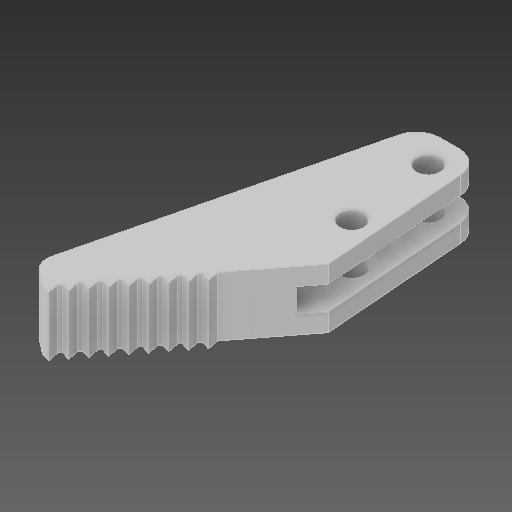
# Autodesk Inventor part: capit
Saved by Autodesk Inventor 2019 (Build 230136000, 136)
## iProperties
Created: 2016-12-05
Part Number: capit
Material: Generic
Document SubType Name: Modeling
Designer: MuhammadArdian
Density: 1 g/cm^3
Appearance: Default
Author: MuhammadArdian
Autodesk Inventor part; units mm, degrees
ref_plane "YZ Plane" through (0, 0, 0) normal (1, 0, 0) x (0, 1, 0)
ref_plane "XZ Plane" through (0, 0, 0) normal (0, 1, 0) x (-1, 0, 0)
sketch "Sketch1" plane through (0, 0, 0) normal (0, 1, 0) x (-1, 0, 0)
  line L0 (-38.3993, -26.9176) -> (-33.0009, -96.7091)
  line L1 (-33.0009, -96.7091) -> (-8.0012, -96.5869)
  circle A0 centre (-23.2715, -84.2034) radius 5
  circle A1 centre (-27.3538, -47.8392) radius 5
  line L2 (-38.3993, -26.9176) -> (16.6007, -26.9176) construction
  arc A2 (22.7463, 28.593) -> (19.9992, 36.438) centre (15.3555, 30.4084) ccw
  line L3 (-8.0012, -96.5869) -> (22.7463, 28.593)
  line L4 (11.975, 39.0871) -> (13.9695, 41.0816)
  line L5 (13.9695, 41.0816) -> (19.9992, 36.438)
  line L6 (13.9695, 41.0816) -> (16.437, 44.2856)
  line L7 (16.437, 44.2856) -> (13.9695, 41.0816)
  line L8 (13.9695, 41.0816) -> (10.2037, 42.2949)
  line L9 (10.2037, 42.2949) -> (11.1441, 37.4129)
  line L10 (10.3086, 36.328) -> (6.5427, 37.5413)
  line L11 (6.5427, 37.5413) -> (7.4831, 32.6592)
  line L12 (6.6476, 31.5743) -> (2.8817, 32.7876)
  line L13 (2.8817, 32.7876) -> (3.8221, 27.9055)
  line L14 (2.9866, 26.8207) -> (-0.7792, 28.034)
  line L15 (-0.7792, 28.034) -> (0.1612, 23.1519)
  line L16 (-0.6744, 22.067) -> (-4.4402, 23.2803)
  line L17 (-4.4402, 23.2803) -> (-3.4998, 18.3982)
  line L18 (-4.3353, 17.3133) -> (-8.1012, 18.5266)
  line L19 (-8.1012, 18.5266) -> (-7.1608, 13.6446)
  line L20 (-7.9963, 12.5597) -> (-11.7622, 13.773)
  line L21 (-11.7622, 13.773) -> (-10.8218, 8.8909)
  line L22 (-11.6573, 7.806) -> (-15.4231, 9.0193)
  line L23 (-15.4231, 9.0193) -> (-14.4827, 4.1373)
  line L24 (-15.3183, 3.0524) -> (-19.0841, 4.2657)
  line L25 (-19.0841, 4.2657) -> (-18.1437, -0.6164)
  line L26 (10.3086, 36.328) -> (11.1441, 37.4129)
  line L27 (6.6476, 31.5743) -> (7.4831, 32.6592)
  line L28 (2.9866, 26.8207) -> (3.8221, 27.9055)
  line L29 (-0.6744, 22.067) -> (0.1612, 23.1519)
  line L30 (-4.3353, 17.3133) -> (-3.4998, 18.3982)
  line L31 (-7.9963, 12.5597) -> (-7.1608, 13.6446)
  line L32 (-11.6573, 7.806) -> (-10.8218, 8.8909)
  line L33 (-38.3993, -26.9176) -> (-18.1437, -0.6164)
  line L34 (-15.3183, 3.0524) -> (-14.4827, 4.1373)
  point P0 (0, 0)
  dimension "d33" = 10
  dimension "d34" = 10
  dimension "d39" = 6
  dimension "d49" = 70
  dimension "d50" = 25
  constraints: 70 end point, 11 tangent, 3 centre point, 2 point on circle, 1 horizontal, 1 perpendicular, 41 other
  measures "d33" diameter of A0
  measures "d34" diameter of A1
  measures "d39" distance of L4.end L10.start
  measures "d49" distance of L0.start L0.end
  measures "d50" distance of L0.end L1.end
extrude "Extrusion3" add sketch "Sketch1" along normal blind 25
ref_plane "Work Plane2" through (0, 12.5, 0) normal (0, 1, 0) x (1, 0, 0)
sketch "Sketch4" plane through (0, 12.5, 0) normal (0, 1, 0) x (1, 0, 0)
  line L0 (41.2703, 100.0732) -> (11.3509, 100.0732)
  line L1 (11.3509, 100.0732) -> (11.3509, 24.6286)
  line L2 (11.3509, 24.6286) -> (41.2703, 17.4466)
  line L3 (41.2703, 17.4466) -> (41.2703, 100.0732)
  point P0 (0, 0)
  constraints: 8 end point, 1 horizontal, 1 perpendicular
extrude "Extrusion4" cut sketch "Sketch4" along normal mid plane 10
fillet "Fillet5" radius 10 4 edges at (33.0009, 21.25, -96.7091) (33.0009, 3.75, -96.7091) (8.0012, 12.5, -96.5869) (11.3509, 12.5, -24.6286)
body "Solid2"
